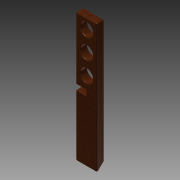
# Autodesk Inventor part: stand1
Saved by Autodesk Inventor 2015 (Build 190159000, 159)
## iProperties
Created: 2014-07-19
Part Number: stand1
Material: Wood (Walnut)
Document SubType Name: Modeling
Designer: pc
Density: 0.55 g/cm^3
Appearance: Walnut - Natural Polished
Author: pc
Autodesk Inventor part; units mm, degrees
ref_plane "YZ Plane" through (0, 0, 0) normal (1, 0, 0) x (0, 1, 0)
ref_plane "XZ Plane" through (0, 0, 0) normal (0, 1, 0) x (-1, 0, 0)
ref_plane "XY Plane" through (0, 0, 0) normal (0, 0, 1) x (1, 0, 0)
sketch "Sketch1" plane through (0, 0, 0) normal (0, 1, 0) x (-1, 0, 0)
  line L0 (21, 130) -> (-21, 130)
  line L1 (-21, 130) -> (-21, -130)
  line L2 (-21, -130) -> (21, -130)
  line L3 (21, -130) -> (21, 130)
  line L4 (21, 130) -> (-21, -130) construction
  line L5 (-21, 130) -> (21, -130) construction
  point P0 (0, 0)
  dimension "d0" = 260
  dimension "d1" = 42
  constraints: 12 end point, 2 midpoint, 2 parallel, 1 horizontal, 1 perpendicular
  measures "d0" distance of L0.end L1.end
  measures "d1" distance of L0.start L0.end
extrude "Extrusion1" add sketch "Sketch1" along normal blind 15
fillet "Fillet4" radius 2 3 edges at (-21, 0, 0) (-21, 7.5, 130) (-21, 15, 0)
sketch "Sketch2" plane through (0, 0, 0) normal (0, -1, 0) x (1, 0, 0)
  circle A0 centre (0, 110) radius 12.5
  circle A1 centre (0, 70) radius 12.5
  circle A2 centre (0, 30) radius 12.5
  line L0 (0, 70) -> (0, 30) construction
  line L1 (0, 110) -> (0, 70) construction
  line L2 (0, 0) -> (0, 148) construction
  line L3 (-37.2491, 0) -> (25.3031, 0) construction
  line L4 (0, -6) -> (-21, -6)
  line L5 (-21, -6) -> (-21, 6)
  line L6 (-21, 6) -> (0, 6)
  line L7 (0, 6) -> (0, -6)
  line L8 (0, -6) -> (-21, 6) construction
  line L9 (-21, -6) -> (0, 6) construction
  line L10 (-21, 128) -> (-21, -130) projected
  line L11 (-19, 130) -> (21, 130) projected
  point P0 (0, 90)
  point P1 (-11.5, 0)
  point P2 (-10.5, 0)
  point P3 (-25, -148)
  point P4 (-21, -130)
  dimension "d9" = 25
  dimension "d10" = 25
  dimension "d11" = 25
  dimension "d12" = 40
  dimension "d13" = 40
  dimension "d16" = 12
  dimension "d36" = 20
  constraints: 20 end point, 3 centre point, 3 midpoint, 3 point on line, 3 vertical, 2 horizontal, 2 parallel, 1 coincident, 1 collinear, 1 perpendicular, 1 other
  measures "d9" diameter of A0
  measures "d10" diameter of A1
  measures "d11" diameter of A2
  measures "d12" distance of L0.start L1.start
  measures "d13" distance of A2.centre L0.start
  measures "d16" distance between parallel lines of L4 L6
  measures "d36" distance from line of L11 L1.start
extrude "Extrusion3" cut sketch "Sketch2" against normal through all
fillet "Fillet6" radius 2 1 edges at (-12.5, 0, 30)
fillet "Fillet7" radius 2 1 edges at (-12.5, 0, 70)
fillet "Fillet8" radius 2 1 edges at (-12.5, 0, 110)
fillet "Fillet9" radius 2 1 edges at (-12.5, 15, 110)
fillet "Fillet10" radius 2 1 edges at (-12.5, 15, 70)
fillet "Fillet11" radius 2 1 edges at (-12.5, 15, 30)
sketch "Sketch4" plane through (21, 0, 130) normal (1, 0, 0) x (0, 0, -1)
  line L0 (260, 0) -> (245, 15)
  line L1 (0, 15) -> (260, 15) projected
  line L2 (260, 0) -> (260, 15)
  point P0 (130, 0)
  dimension "d29" = 45
  constraints: 4 end point, 1 perpendicular, 1 point on line
  measures "d29" angle of L1 L0
extrude "Extrusion4" cut sketch "Sketch4" against normal through all
fillet "Fillet12" radius 2 1 edges at (21, 0, 0)
fillet "Fillet13" radius 2 1 edges at (21, 15, 7.5)
fillet "Fillet14" radius 2 8 edges at (21, 7.5, -122.5) (20.4142, 14.4142, -115.5858) (0, 15, -115) (-20.4142, 14.4142, -115.5858) (-21, 7.5, -122.5) (-20.4142, 0.5858, -129.4142) (0, 0, -130) (20.4142, 0.5858, -129.4142)
fillet "Fillet15" radius 2 7 edges at (21, 7.5, 130) (20.4142, 14.4142, 130) (0, 15, 130) (-20.4142, 14.4142, 129.4142) (20.4142, 0.5858, 130) (0, 0, 130) (-20.4142, 0.5858, 129.4142)
equation "\"d13\" = d12"
body "Solid1"
